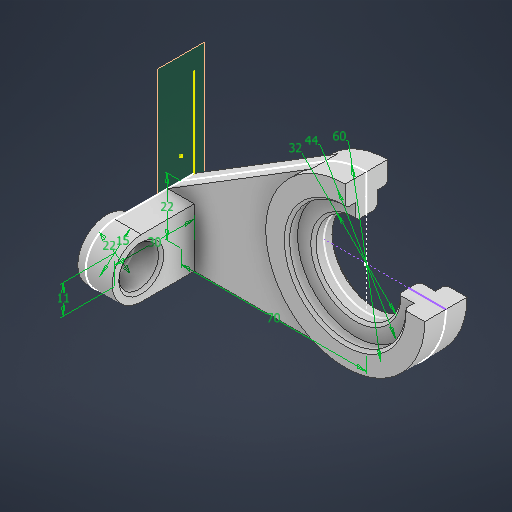
# Autodesk Inventor part: Day02_Task02
Saved by Autodesk Inventor 2027.1 (Build 311270010, 270A)
## iProperties
Created: 2026-08-05
Part Number: Day02_Task02
Material: 일반
Document SubType Name: Modeling
Designer: lkh06
Density: 1 g/cm^3
Appearance: 기본값
Author: lkh06
Autodesk Inventor part; units mm, degrees
ref_plane "YZ Plane" through (0, 0, 0) normal (1, 0, 0) x (0, 1, 0)
ref_plane "XZ Plane" through (0, 0, 0) normal (0, 1, 0) x (-1, 0, 0)
ref_plane "XY Plane" through (0, 0, 0) normal (0, 0, 1) x (1, 0, 0)
sketch "스케치1" plane through (0, 0, 0) normal (0, 0, 1) x (1, 0, 0)
  arc A0 (0, 16) -> (16, 0) centre (0, 0) ccw
  arc A1 (0, 22) -> (22, 0) centre (0, 0) ccw
  arc A2 (0, 30) -> (30, 0) centre (0, 0) ccw
  line L0 (0, -30) -> (-70, -30)
  line L1 (-70, -30) -> (-70, -8)
  line L2 (-70, -8) -> (-15.7735, 25.5185)
  line L3 (0, -30) -> (0, 30) construction
  line L4 (-30, 0) -> (30, 0) construction
  line L5 (0, 30) -> (0, 16)
  line L6 (16, 0) -> (30, 0)
  point P0 (0, 22)
  point P1 (22, 0)
  dimension "d0" = 32
  dimension "d1" = 44
  dimension "d2" = 60
  dimension "d3" = 70
  dimension "d4" = 22
  constraints: 14 end point, 9 point on circle, 4 point on line, 3 centre point, 3 coincident, 2 collinear, 2 perpendicular, 2 tangent, 1 horizontal, 1 vertical
  measures "d0" diameter of A0
  measures "d1" diameter of A1
  measures "d2" diameter of A2
  measures "d3" distance of L0.start L0.end
  measures "d4" distance of L0.end L1.end
extrude "돌출1" add sketch "스케치1" along normal blind 4 contours A0 L6 A1 L5
extrude "돌출2" add sketch "스케치1" along normal blind 8 contours A1 L6 A2 L5
extrude "돌출3" add sketch "스케치1" along normal blind 5 contours A2 L0 L1 L2
chamfer "모따기1" distance 1 angle 45 1 edges at (-15.5563, -15.5563, 8)
chamfer "모따기2" distance 1 angle 45 1 edges at (-11.3137, -11.3137, 4)
mirror "미러1" about plane through (0, 0, 0) normal (0, 0, -1)
ref_plane "작업 평면1" through (-70, -30, 0) normal (-1, 0, 0) x (0, 0, 1)
sketch "스케치2" plane through (-70, -30, 0) normal (-1, 0, 0) x (0, 0, 1)
  line L0 (-5, 0) -> (-5, 55.5185) projected
  line L1 (-5, 0) -> (25, 0)
  circle A0 centre (25, 11) radius 7.5
  circle A1 centre (25, 11) radius 11
  line L2 (25, 22) -> (-5, 22)
  line L3 (-5, 22) -> (-5, 0) projected
  line L4 (25, 0) -> (25, 22) construction
  point P0 (0, 30)
  dimension "d17" = 30
  dimension "d21" = 11
  dimension "d22" = 15
  dimension "d23" = 22
  constraints: 6 end point, 2 centre point, 2 perpendicular, 2 point on line, 1 coincident, 1 horizontal, 1 midpoint, 1 parallel, 1 tangent
  measures "d17" distance of L0.start L1.end
  measures "d21" distance of L1.end A0.centre
  measures "d22" diameter of A0
  measures "d23" diameter of A1
extrude "돌출4" add sketch "스케치2" against normal blind 10 contours L0 L2 A1 L1
extrude "돌출5" add sketch "스케치2" against normal blind 10 contours A1
extrude "돌출6" add sketch "스케치2" along normal blind 3 contours A1
chamfer "모따기3" distance 1 angle 45 1 edges at (-73, -19, 17.5)
chamfer "모따기4" distance 1 angle 45 1 edges at (-60, -19, 17.5)
